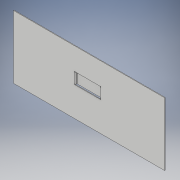
# Autodesk Inventor part: DecupajAgatare1
Saved by Autodesk Inventor 2019 (Build 230136000, 136)
## iProperties
Created: 2020-04-08
Part Number: DecupajAgatare1
Material: Generic
Document SubType Name: Sheet Metal
Designer: Gabriel
Density: 1 g/cm^3
Sheet Metal Rule: Default_mm
Appearance: Default
Author: Gabriel
Autodesk Inventor part; units mm, degrees
ref_plane "YZ Plane" through (0, 0, 0) normal (1, 0, 0) x (0, 1, 0)
ref_plane "XZ Plane" through (0, 0, 0) normal (0, 1, 0) x (-1, 0, 0)
ref_plane "XY Plane" through (0, 0, 0) normal (0, 0, 1) x (1, 0, 0)
sketch "Sketch1" plane through (0, 0, 0) normal (0, 0, 1) x (1, 0, 0)
  line L0 (-61.6808, 42.3688) -> (58.3192, 42.3688)
  line L1 (58.3192, 42.3688) -> (58.3192, -7.6312)
  line L2 (58.3192, -7.6312) -> (-61.6808, -7.6312)
  line L3 (-61.6808, -7.6312) -> (-61.6808, 42.3688)
  dimension "d0" = 50
  dimension "d1" = 120
  measures "d0" distance of L0.end L1.end
  measures "d1" distance of L1.end L2.end
extrude "Plate1" add sketch "Sketch1" along normal blind 0.5
sketch "Sketch2" plane through (0, 0, 0.5) normal (0, 0, 1) x (1, 0, 0)
  line L0 (-12.7986, 24.2423) -> (7.2014, 24.2423)
  line L1 (7.2014, 24.2423) -> (7.2014, 16.2423)
  line L2 (7.2014, 16.2423) -> (-12.7986, 16.2423)
  line L3 (-12.7986, 16.2423) -> (-12.7986, 24.2423)
  point P0 (-2.7986, 20.2423)
  dimension "LG_G" = 20
  dimension "LT_G" = 8
  dimension "d21" = 4
  dimension "d22" = 10
  constraints: 8 end point, 2 parallel, 1 horizontal, 1 perpendicular, 1 vertical alignment
  measures "LG_G" distance of L0.start L0.end
  measures "LT_G" distance of L0.end L1.end
  measures "d21" distance from line of L0 point (-2.799, 20.242)
  measures "d22" distance from line of L3 point (-2.799, 20.242)
extrude "Extrusion1" add sketch "Sketch2" against normal blind 1.5
sketch "Sketch3" plane through (0, 0, 0.5) normal (0, 0, 1) x (1, 0, 0)
  line L0 (-12.7986, 24.2423) -> (7.2014, 24.2423) projected
  line L1 (-12.7986, 16.2423) -> (-12.7986, 24.2423) projected
  line L2 (7.2014, 16.2423) -> (-12.7986, 16.2423) projected
  line L3 (7.2014, 24.2423) -> (7.2014, 16.2423) projected
  line L4 (-12.2986, 24.2423) -> (6.7014, 24.2423)
  line L5 (6.7014, 24.2423) -> (6.7014, 16.2423)
  line L6 (6.7014, 16.2423) -> (-12.2986, 16.2423)
  line L7 (-12.2986, 16.2423) -> (-12.2986, 24.2423)
  dimension "d9" = 0.5
  dimension "d10" = 0.5
  constraints: 8 end point, 2 collinear, 2 parallel, 1 horizontal, 1 perpendicular
  measures "d9" distance of L2.start L5.end
  measures "d10" distance of L1.start L6.end
extrude "Extrusion2" cut sketch "Sketch3" against normal blind 1 contours L0 L5 L2 L7
sketch "Sketch4" plane through (0, 0, 0.5) normal (0, 0, 1) x (1, 0, 0)
  line L0 (-12.7986, 24.2423) -> (7.2014, 24.2423) projected
  line L1 (-12.7986, 16.2423) -> (-12.7986, 24.2423) projected
  line L2 (7.2014, 24.2423) -> (7.2014, 16.2423) projected
  line L3 (7.2014, 16.2423) -> (-12.7986, 16.2423) projected
  line L4 (-13.2986, 24.7423) -> (7.7014, 24.7423)
  line L5 (7.7014, 24.7423) -> (7.7014, 24.2423)
  line L6 (7.7014, 24.2423) -> (-13.2986, 24.2423)
  line L7 (-13.2986, 24.2423) -> (-13.2986, 24.7423)
  line L8 (-13.2986, 16.2423) -> (7.7014, 16.2423)
  line L9 (7.7014, 16.2423) -> (7.7014, 15.7423)
  line L10 (7.7014, 15.7423) -> (-13.2986, 15.7423)
  line L11 (-13.2986, 15.7423) -> (-13.2986, 16.2423)
  line L12 (6.7014, 16.2423) -> (-12.2986, 16.2423) projected
  dimension "d13" = 0.5
  dimension "d14" = 0.5
  dimension "d15" = 0.5
  dimension "d16" = 0.5
  constraints: 16 end point, 4 collinear, 4 parallel, 4 point on line, 2 horizontal, 2 perpendicular
  measures "d13" distance of L10.end L8.start
  measures "d14" distance of L6.end L4.start
  measures "d15" distance of L8.start L1.start
  measures "d16" distance of L8.end L2.end
extrude "Cut1" cut sketch "Sketch4" against normal blind 0.5 contours L6 L7 L4 L5 L0 | L3 L8 L9 L10 L11
fillet "Fillet1" radius 0.8 4 edges at (-12.2986, 20.2423, 0.5) (6.7014, 20.2423, 0.5) (-12.7986, 20.2423, -1) (7.2014, 20.2423, -1)
fillet "Fillet2" radius 0.3 4 edges at (7.2014, 20.2423, 0) (-12.7986, 20.2423, 0) (-12.2986, 20.2423, -0.5) (6.7014, 20.2423, -0.5)
equation "\"d21\" = 0.5 * LT_G"
equation "\"d22\" = 0.5 * LG_G"
equation "\"d7\" = 3 * Thickness"
equation "\"d9\" = Thickness"
equation "\"d10\" = Thickness"
equation "\"d11\" = 2 * Thickness"
equation "\"d13\" = Thickness"
equation "\"d14\" = Thickness"
equation "\"d15\" = Thickness"
equation "\"d16\" = Thickness"
equation "\"d17\" = Thickness"
equation "\"d2\" = Thickness"
equation "\"BendRadius\" = Thickness"
equation "\"BendReliefWidth\" = Thickness"
equation "\"BendReliefDepth\" = 0.5 * Thickness"
equation "\"CornerReliefSize\" = 4 * Thickness"
equation "\"MinimumRemnant\" = 2 * Thickness"
equation "\"TransitionRadius\" = BendRadius"
equation "\"JacobiRadiusSize\" = BendRadius"
equation "\"GapSize\" = Thickness"
equation "\"Thickness\" = 0.5"
body "Solid1"
